Autodesk Fusion 360 part; units mm, degrees
(part 10 of 18)
  line L6698 (176.3253, -58.2178) -> (176.3253, -57.3778)
  line L6699 (176.3253, -57.3778) -> (177.2353, -57.3778)
  line L6700 (180.5454, -57.3778) -> (180.5454, -58.2178)
  line L6701 (180.5454, -58.2178) -> (179.6354, -58.2178)
  line L6702 (179.6354, -58.2178) -> (179.6354, -57.3778)
  line L6703 (179.6354, -57.3778) -> (180.5454, -57.3778)
  line L6704 (176.3253, -38.3151) -> (177.2353, -38.3151)
  line L6705 (177.2353, -39.1551) -> (176.3253, -39.1551)
  line L6706 (176.3253, -39.1551) -> (176.3253, -38.3151)
  line L6707 (177.2353, -38.3151) -> (177.2353, -39.1551)
  line L6708 (180.5454, -39.1551) -> (179.6354, -39.1551)
  line L6709 (180.5454, -38.3151) -> (180.5454, -39.1551)
  line L6710 (179.6354, -38.3151) -> (180.5454, -38.3151)
  line L6711 (179.6354, -39.1551) -> (179.6354, -38.3151)
  line L6712 (100.1251, -77.2806) -> (100.1251, -76.4406)
  line L6713 (100.1251, -76.4406) -> (101.0351, -76.4406)
  line L6714 (101.0351, -77.2806) -> (100.1251, -77.2806)
  line L6715 (101.0351, -76.4406) -> (101.0351, -77.2806)
  line L6716 (104.3453, -77.2806) -> (103.4353, -77.2806)
  line L6717 (104.3453, -76.4406) -> (104.3453, -77.2806)
  line L6718 (103.4353, -76.4406) -> (104.3453, -76.4406)
  line L6719 (103.4353, -77.2806) -> (103.4353, -76.4406)
  line L6720 (100.1251, -57.3778) -> (101.0351, -57.3778)
  line L6721 (101.0351, -58.2178) -> (100.1251, -58.2178)
  line L6722 (100.1251, -58.2178) -> (100.1251, -57.3778)
  line L6723 (101.0351, -57.3778) -> (101.0351, -58.2178)
  line L6724 (104.3453, -58.2178) -> (103.4353, -58.2178)
  line L6725 (104.3453, -57.3778) -> (104.3453, -58.2178)
  line L6726 (103.4353, -58.2178) -> (103.4353, -57.3778)
  line L6727 (103.4353, -57.3778) -> (104.3453, -57.3778)
  line L6728 (100.1251, -19.265) -> (101.0351, -19.265)
  line L6729 (101.0351, -20.105) -> (100.1251, -20.105)
  line L6730 (100.1251, -20.105) -> (100.1251, -19.265)
  line L6731 (101.0351, -19.265) -> (101.0351, -20.105)
  line L6732 (103.4353, -20.105) -> (103.4353, -19.265)
  line L6733 (104.3453, -20.105) -> (103.4353, -20.105)
  line L6734 (104.3453, -19.265) -> (104.3453, -20.105)
  line L6735 (103.4353, -19.265) -> (104.3453, -19.265)
  line L6736 (100.1251, -39.1551) -> (100.1251, -38.3151)
  line L6737 (100.1251, -38.3151) -> (101.0351, -38.3151)
  line L6738 (101.0351, -38.3151) -> (101.0351, -39.1551)
  line L6739 (101.0351, -39.1551) -> (100.1251, -39.1551)
  line L6740 (104.3453, -38.3151) -> (104.3453, -39.1551)
  line L6741 (103.4353, -39.1551) -> (103.4353, -38.3151)
  line L6742 (104.3453, -39.1551) -> (103.4353, -39.1551)
  line L6743 (103.4353, -38.3151) -> (104.3453, -38.3151)
  line L6744 (119.1752, -20.105) -> (119.1752, -19.265)
  line L6745 (120.0852, -20.105) -> (119.1752, -20.105)
  line L6746 (119.1752, -19.265) -> (120.0852, -19.265)
  line L6747 (120.0852, -19.265) -> (120.0852, -20.105)
  line L6748 (122.4853, -19.265) -> (123.3953, -19.265)
  line L6749 (123.3953, -20.105) -> (122.4853, -20.105)
  line L6750 (123.3953, -19.265) -> (123.3953, -20.105)
  line L6751 (122.4853, -20.105) -> (122.4853, -19.265)
  line L6752 (119.1752, -58.2178) -> (119.1752, -57.3778)
  line L6753 (120.0852, -58.2178) -> (119.1752, -58.2178)
  line L6754 (120.0852, -57.3778) -> (120.0852, -58.2178)
  line L6755 (119.1752, -57.3778) -> (120.0852, -57.3778)
  line L6756 (122.4853, -58.2178) -> (122.4853, -57.3778)
  line L6757 (123.3953, -57.3778) -> (123.3953, -58.2178)
  line L6758 (123.3953, -58.2178) -> (122.4853, -58.2178)
  line L6759 (122.4853, -57.3778) -> (123.3953, -57.3778)
  line L6760 (120.0852, -38.3151) -> (120.0852, -39.1551)
  line L6761 (119.1752, -38.3151) -> (120.0852, -38.3151)
  line L6762 (119.1752, -39.1551) -> (119.1752, -38.3151)
  line L6763 (120.0852, -39.1551) -> (119.1752, -39.1551)
  line L6764 (123.3953, -38.3151) -> (123.3953, -39.1551)
  line L6765 (123.3953, -39.1551) -> (122.4853, -39.1551)
  line L6766 (122.4853, -39.1551) -> (122.4853, -38.3151)
  line L6767 (122.4853, -38.3151) -> (123.3953, -38.3151)
  line L6768 (120.0852, -77.2806) -> (119.1752, -77.2806)
  line L6769 (119.1752, -77.2806) -> (119.1752, -76.4406)
  line L6770 (119.1752, -76.4406) -> (120.0852, -76.4406)
  line L6771 (120.0852, -76.4406) -> (120.0852, -77.2806)
  line L6772 (123.3953, -77.2806) -> (122.4853, -77.2806)
  line L6773 (123.3953, -76.4406) -> (123.3953, -77.2806)
  line L6774 (122.4853, -76.4406) -> (123.3953, -76.4406)
  line L6775 (122.4853, -77.2806) -> (122.4853, -76.4406)
  line L6776 (5.785, -76.4406) -> (5.785, -77.2806)
  line L6777 (5.785, -77.2806) -> (4.8749, -77.2806)
  line L6778 (4.8749, -76.4406) -> (5.785, -76.4406)
  line L6779 (4.8749, -77.2806) -> (4.8749, -76.4406)
  line L6780 (9.0951, -76.4406) -> (9.0951, -77.2806)
  line L6781 (8.1851, -76.4406) -> (9.0951, -76.4406)
  line L6782 (8.1851, -77.2806) -> (8.1851, -76.4406)
  line L6783 (9.0951, -77.2806) -> (8.1851, -77.2806)
  line L6784 (23.925, -76.4406) -> (24.835, -76.4406)
  line L6785 (23.925, -77.2806) -> (23.925, -76.4406)
  line L6786 (24.835, -77.2806) -> (23.925, -77.2806)
  line L6787 (24.835, -76.4406) -> (24.835, -77.2806)
  line L6788 (28.1451, -76.4406) -> (28.1451, -77.2806)
  line L6789 (28.1451, -77.2806) -> (27.2351, -77.2806)
  line L6790 (27.2351, -77.2806) -> (27.2351, -76.4406)
  line L6791 (27.2351, -76.4406) -> (28.1451, -76.4406)
  line L6792 (42.975, -76.4406) -> (43.885, -76.4406)
  line L6793 (42.975, -77.2806) -> (42.975, -76.4406)
  line L6794 (43.885, -77.2806) -> (42.975, -77.2806)
  line L6795 (43.885, -76.4406) -> (43.885, -77.2806)
  line L6796 (46.2852, -77.2806) -> (46.2852, -76.4406)
  line L6797 (47.1952, -76.4406) -> (47.1952, -77.2806)
  line L6798 (47.1952, -77.2806) -> (46.2852, -77.2806)
  line L6799 (46.2852, -76.4406) -> (47.1952, -76.4406)
  line L6800 (62.0251, -19.265) -> (62.9351, -19.265)
  line L6801 (62.0251, -20.105) -> (62.0251, -19.265)
  line L6802 (62.9351, -20.105) -> (62.0251, -20.105)
  line L6803 (62.9351, -19.265) -> (62.9351, -20.105)
  line L6804 (65.3352, -20.105) -> (65.3352, -19.265)
  line L6805 (65.3352, -19.265) -> (66.2452, -19.265)
  line L6806 (66.2452, -20.105) -> (65.3352, -20.105)
  line L6807 (66.2452, -19.265) -> (66.2452, -20.105)
  line L6808 (62.0251, -76.4406) -> (62.9351, -76.4406)
  line L6809 (62.0251, -77.2806) -> (62.0251, -76.4406)
  line L6810 (62.9351, -76.4406) -> (62.9351, -77.2806)
  line L6811 (62.9351, -77.2806) -> (62.0251, -77.2806)
  line L6812 (65.3352, -76.4406) -> (66.2452, -76.4406)
  line L6813 (66.2452, -76.4406) -> (66.2452, -77.2806)
  line L6814 (66.2452, -77.2806) -> (65.3352, -77.2806)
  line L6815 (65.3352, -77.2806) -> (65.3352, -76.4406)
  line L6816 (62.0251, -38.3151) -> (62.9351, -38.3151)
  line L6817 (62.9351, -38.3151) -> (62.9351, -39.1551)
  line L6818 (62.0251, -39.1551) -> (62.0251, -38.3151)
  line L6819 (62.9351, -39.1551) -> (62.0251, -39.1551)
  line L6820 (66.2452, -38.3151) -> (66.2452, -39.1551)
  line L6821 (66.2452, -39.1551) -> (65.3352, -39.1551)
  line L6822 (65.3352, -38.3151) -> (66.2452, -38.3151)
  line L6823 (65.3352, -39.1551) -> (65.3352, -38.3151)
  line L6824 (62.9351, -58.2178) -> (62.0251, -58.2178)
  line L6825 (62.0251, -57.3778) -> (62.9351, -57.3778)
  line L6826 (62.0251, -58.2178) -> (62.0251, -57.3778)
  line L6827 (62.9351, -57.3778) -> (62.9351, -58.2178)
  line L6828 (66.2452, -57.3778) -> (66.2452, -58.2178)
  line L6829 (65.3352, -57.3778) -> (66.2452, -57.3778)
  line L6830 (66.2452, -58.2178) -> (65.3352, -58.2178)
  line L6831 (65.3352, -58.2178) -> (65.3352, -57.3778)
  line L6832 (81.9851, -39.1551) -> (81.0751, -39.1551)
  line L6833 (81.0751, -38.3151) -> (81.9851, -38.3151)
  line L6834 (81.9851, -38.3151) -> (81.9851, -39.1551)
  line L6835 (81.0751, -39.1551) -> (81.0751, -38.3151)
  line L6836 (84.3852, -38.3151) -> (85.2952, -38.3151)
  line L6837 (85.2952, -39.1551) -> (84.3852, -39.1551)
  line L6838 (84.3852, -39.1551) -> (84.3852, -38.3151)
  line L6839 (85.2952, -38.3151) -> (85.2952, -39.1551)
  line L6840 (81.9851, -77.2806) -> (81.0751, -77.2806)
  line L6841 (81.9851, -76.4406) -> (81.9851, -77.2806)
  line L6842 (81.0751, -77.2806) -> (81.0751, -76.4406)
  line L6843 (81.0751, -76.4406) -> (81.9851, -76.4406)
  line L6844 (84.3852, -76.4406) -> (85.2952, -76.4406)
  line L6845 (85.2952, -77.2806) -> (84.3852, -77.2806)
  line L6846 (84.3852, -77.2806) -> (84.3852, -76.4406)
  line L6847 (85.2952, -76.4406) -> (85.2952, -77.2806)
  line L6848 (81.9851, -19.265) -> (81.9851, -20.105)
  line L6849 (81.9851, -20.105) -> (81.0751, -20.105)
  line L6850 (81.0751, -19.265) -> (81.9851, -19.265)
  line L6851 (81.0751, -20.105) -> (81.0751, -19.265)
  line L6852 (85.2952, -19.265) -> (85.2952, -20.105)
  line L6853 (84.3852, -19.265) -> (85.2952, -19.265)
  line L6854 (84.3852, -20.105) -> (84.3852, -19.265)
  line L6855 (85.2952, -20.105) -> (84.3852, -20.105)
  line L6856 (81.9851, -58.2178) -> (81.0751, -58.2178)
  line L6857 (81.0751, -57.3778) -> (81.9851, -57.3778)
  line L6858 (81.9851, -57.3778) -> (81.9851, -58.2178)
  line L6859 (81.0751, -58.2178) -> (81.0751, -57.3778)
  line L6860 (84.3852, -58.2178) -> (84.3852, -57.3778)
  line L6861 (85.2952, -57.3778) -> (85.2952, -58.2178)
  line L6862 (84.3852, -57.3778) -> (85.2952, -57.3778)
  line L6863 (85.2952, -58.2178) -> (84.3852, -58.2178)
  line L6864 (5.785, -58.2178) -> (4.8749, -58.2178)
  line L6865 (5.785, -57.3778) -> (5.785, -58.2178)
  line L6866 (4.8749, -57.3778) -> (5.785, -57.3778)
  line L6867 (4.8749, -58.2178) -> (4.8749, -57.3778)
  line L6868 (8.1851, -58.2178) -> (8.1851, -57.3778)
  line L6869 (8.1851, -57.3778) -> (9.0951, -57.3778)
  line L6870 (9.0951, -57.3778) -> (9.0951, -58.2178)
  line L6871 (9.0951, -58.2178) -> (8.1851, -58.2178)
  line L6872 (4.8749, -19.265) -> (5.785, -19.265)
  line L6873 (5.785, -20.105) -> (4.8749, -20.105)
  line L6874 (5.785, -19.265) -> (5.785, -20.105)
  line L6875 (4.8749, -20.105) -> (4.8749, -19.265)
  line L6876 (8.1851, -20.105) -> (8.1851, -19.265)
  line L6877 (9.0951, -20.105) -> (8.1851, -20.105)
  line L6878 (8.1851, -19.265) -> (9.0951, -19.265)
  line L6879 (9.0951, -19.265) -> (9.0951, -20.105)
  line L6880 (4.8749, -39.1551) -> (4.8749, -38.3151)
  line L6881 (5.785, -38.3151) -> (5.785, -39.1551)
  line L6882 (5.785, -39.1551) -> (4.8749, -39.1551)
  line L6883 (4.8749, -38.3151) -> (5.785, -38.3151)
  line L6884 (9.0951, -38.3151) -> (9.0951, -39.1551)
  line L6885 (8.1851, -39.1551) -> (8.1851, -38.3151)
  line L6886 (9.0951, -39.1551) -> (8.1851, -39.1551)
  line L6887 (8.1851, -38.3151) -> (9.0951, -38.3151)
  line L6888 (24.835, -38.3151) -> (24.835, -39.1551)
  line L6889 (24.835, -39.1551) -> (23.925, -39.1551)
  line L6890 (23.925, -39.1551) -> (23.925, -38.3151)
  line L6891 (23.925, -38.3151) -> (24.835, -38.3151)
  line L6892 (27.2351, -39.1551) -> (27.2351, -38.3151)
  line L6893 (28.1451, -39.1551) -> (27.2351, -39.1551)
  line L6894 (27.2351, -38.3151) -> (28.1451, -38.3151)
  line L6895 (28.1451, -38.3151) -> (28.1451, -39.1551)
  line L6896 (24.835, -19.265) -> (24.835, -20.105)
  line L6897 (23.925, -20.105) -> (23.925, -19.265)
  line L6898 (24.835, -20.105) -> (23.925, -20.105)
  line L6899 (23.925, -19.265) -> (24.835, -19.265)
  line L6900 (27.2351, -20.105) -> (27.2351, -19.265)
  line L6901 (28.1451, -19.265) -> (28.1451, -20.105)
  line L6902 (28.1451, -20.105) -> (27.2351, -20.105)
  line L6903 (27.2351, -19.265) -> (28.1451, -19.265)
  line L6904 (23.925, -58.2178) -> (23.925, -57.3778)
  line L6905 (24.835, -58.2178) -> (23.925, -58.2178)
  line L6906 (23.925, -57.3778) -> (24.835, -57.3778)
  line L6907 (24.835, -57.3778) -> (24.835, -58.2178)
  line L6908 (28.1451, -58.2178) -> (27.2351, -58.2178)
  line L6909 (28.1451, -57.3778) -> (28.1451, -58.2178)
  line L6910 (27.2351, -57.3778) -> (28.1451, -57.3778)
  line L6911 (27.2351, -58.2178) -> (27.2351, -57.3778)
  line L6912 (43.885, -19.265) -> (43.885, -20.105)
  line L6913 (42.975, -19.265) -> (43.885, -19.265)
  line L6914 (42.975, -20.105) -> (42.975, -19.265)
  line L6915 (43.885, -20.105) -> (42.975, -20.105)
  line L6916 (47.1952, -20.105) -> (46.2852, -20.105)
  line L6917 (47.1952, -19.265) -> (47.1952, -20.105)
  line L6918 (46.2852, -19.265) -> (47.1952, -19.265)
  line L6919 (46.2852, -20.105) -> (46.2852, -19.265)
  line L6920 (43.885, -57.3778) -> (43.885, -58.2178)
  line L6921 (42.975, -57.3778) -> (43.885, -57.3778)
  line L6922 (42.975, -58.2178) -> (42.975, -57.3778)
  line L6923 (43.885, -58.2178) -> (42.975, -58.2178)
  line L6924 (46.2852, -57.3778) -> (47.1952, -57.3778)
  line L6925 (47.1952, -57.3778) -> (47.1952, -58.2178)
  line L6926 (46.2852, -58.2178) -> (46.2852, -57.3778)
  line L6927 (47.1952, -58.2178) -> (46.2852, -58.2178)
  line L6928 (43.885, -38.3151) -> (43.885, -39.1551)
  line L6929 (42.975, -38.3151) -> (43.885, -38.3151)
  line L6930 (43.885, -39.1551) -> (42.975, -39.1551)
  line L6931 (42.975, -39.1551) -> (42.975, -38.3151)
  line L6932 (47.1952, -38.3151) -> (47.1952, -39.1551)
  line L6933 (46.2852, -39.1551) -> (46.2852, -38.3151)
  line L6934 (47.1952, -39.1551) -> (46.2852, -39.1551)
  line L6935 (46.2852, -38.3151) -> (47.1952, -38.3151)
  line L6936 (215.3354, -20.105) -> (214.4254, -20.105)
  line L6937 (214.4254, -19.265) -> (215.3354, -19.265)
  line L6938 (214.4254, -20.105) -> (214.4254, -19.265)
  line L6939 (215.3354, -19.265) -> (215.3354, -20.105)
  line L6940 (218.6455, -19.265) -> (218.6455, -20.105)
  line L6941 (217.7355, -20.105) -> (217.7355, -19.265)
  line L6942 (218.6455, -20.105) -> (217.7355, -20.105)
  line L6943 (217.7355, -19.265) -> (218.6455, -19.265)
  line L6944 (215.3354, -76.4406) -> (215.3354, -77.2806)
  line L6945 (214.4254, -76.4406) -> (215.3354, -76.4406)
  line L6946 (214.4254, -77.2806) -> (214.4254, -76.4406)
  line L6947 (215.3354, -77.2806) -> (214.4254, -77.2806)
  line L6948 (218.6455, -77.2806) -> (217.7355, -77.2806)
  line L6949 (217.7355, -77.2806) -> (217.7355, -76.4406)
  line L6950 (218.6455, -76.4406) -> (218.6455, -77.2806)
  line L6951 (217.7355, -76.4406) -> (218.6455, -76.4406)
  line L6952 (214.4254, -57.3778) -> (215.3354, -57.3778)
  line L6953 (214.4254, -58.2178) -> (214.4254, -57.3778)
  line L6954 (215.3354, -58.2178) -> (214.4254, -58.2178)
  line L6955 (215.3354, -57.3778) -> (215.3354, -58.2178)
  line L6956 (217.7355, -58.2178) -> (217.7355, -57.3778)
  line L6957 (217.7355, -57.3778) -> (218.6455, -57.3778)
  line L6958 (218.6455, -58.2178) -> (217.7355, -58.2178)
  line L6959 (218.6455, -57.3778) -> (218.6455, -58.2178)
  line L6960 (214.4254, -38.3151) -> (215.3354, -38.3151)
  line L6961 (214.4254, -39.1551) -> (214.4254, -38.3151)
  line L6962 (215.3354, -39.1551) -> (214.4254, -39.1551)
  line L6963 (215.3354, -38.3151) -> (215.3354, -39.1551)
  line L6964 (217.7355, -39.1551) -> (217.7355, -38.3151)
  line L6965 (218.6455, -38.3151) -> (218.6455, -39.1551)
  line L6966 (218.6455, -39.1551) -> (217.7355, -39.1551)
  line L6967 (217.7355, -38.3151) -> (218.6455, -38.3151)
  line L6968 (196.2853, -38.3151) -> (196.2853, -39.1551)
  line L6969 (195.3753, -39.1551) -> (195.3753, -38.3151)
  line L6970 (196.2853, -39.1551) -> (195.3753, -39.1551)
  line L6971 (195.3753, -38.3151) -> (196.2853, -38.3151)
  line L6972 (199.5955, -38.3151) -> (199.5955, -39.1551)
  line L6973 (198.6855, -39.1551) -> (198.6855, -38.3151)
  line L6974 (199.5955, -39.1551) -> (198.6855, -39.1551)
  line L6975 (198.6855, -38.3151) -> (199.5955, -38.3151)
  line L6976 (195.3753, -76.4406) -> (196.2853, -76.4406)
  line L6977 (196.2853, -76.4406) -> (196.2853, -77.2806)
  line L6978 (196.2853, -77.2806) -> (195.3753, -77.2806)
  line L6979 (195.3753, -77.2806) -> (195.3753, -76.4406)
  line L6980 (199.5955, -77.2806) -> (198.6855, -77.2806)
  line L6981 (198.6855, -76.4406) -> (199.5955, -76.4406)
  line L6982 (198.6855, -77.2806) -> (198.6855, -76.4406)
  line L6983 (199.5955, -76.4406) -> (199.5955, -77.2806)
  line L6984 (196.2853, -58.2178) -> (195.3753, -58.2178)
  line L6985 (195.3753, -57.3778) -> (196.2853, -57.3778)
  line L6986 (195.3753, -58.2178) -> (195.3753, -57.3778)
  line L6987 (196.2853, -57.3778) -> (196.2853, -58.2178)
  line L6988 (199.5955, -57.3778) -> (199.5955, -58.2178)
  line L6989 (198.6855, -58.2178) -> (198.6855, -57.3778)
  line L6990 (198.6855, -57.3778) -> (199.5955, -57.3778)
  line L6991 (199.5955, -58.2178) -> (198.6855, -58.2178)
  line L6992 (196.2853, -19.265) -> (196.2853, -20.105)
  line L6993 (195.3753, -20.105) -> (195.3753, -19.265)
  line L6994 (196.2853, -20.105) -> (195.3753, -20.105)
  line L6995 (195.3753, -19.265) -> (196.2853, -19.265)
  line L6996 (199.5955, -19.265) -> (199.5955, -20.105)
  line L6997 (198.6855, -20.105) -> (198.6855, -19.265)
  line L6998 (198.6855, -19.265) -> (199.5955, -19.265)
  line L6999 (199.5955, -20.105) -> (198.6855, -20.105)
  line L7000 (202.1384, -4.26) -> (201.3384, -4.26)
  line L7001 (202.1384, -3.36) -> (202.1384, -4.26)
  line L7002 (201.3384, -3.36) -> (202.1384, -3.36)
  line L7003 (201.3384, -4.26) -> (201.3384, -3.36)
  line L7004 (202.7384, -3.36) -> (203.5384, -3.36)
  line L7005 (203.5384, -3.36) -> (203.5384, -4.26)
  line L7006 (202.7384, -4.26) -> (202.7384, -3.36)
  line L7007 (203.5384, -4.26) -> (202.7384, -4.26)
  line L7008 (200.2334, -6.281) -> (200.2334, -7.181)
  line L7009 (200.2334, -7.181) -> (199.4334, -7.181)
  line L7010 (199.4334, -6.281) -> (200.2334, -6.281)
  line L7011 (199.4334, -7.181) -> (199.4334, -6.281)
  line L7012 (201.6334, -7.181) -> (200.8334, -7.181)
  line L7013 (200.8334, -6.281) -> (201.6334, -6.281)
  line L7014 (201.6334, -6.281) -> (201.6334, -7.181)
  line L7015 (200.8334, -7.181) -> (200.8334, -6.281)
  line L7016 (206.8404, -4.376) -> (206.8404, -5.276)
  line L7017 (206.8404, -5.276) -> (206.0404, -5.276)
  line L7018 (206.0404, -4.376) -> (206.8404, -4.376)
  line L7019 (206.0404, -5.276) -> (206.0404, -4.376)
  line L7020 (205.4404, -4.376) -> (205.4404, -5.276)
  line L7021 (204.6404, -5.276) -> (204.6404, -4.376)
  line L7022 (204.6404, -4.376) -> (205.4404, -4.376)
  line L7023 (205.4404, -5.276) -> (204.6404, -5.276)
  arc A868 (8.7631, -8.0011) -> (10.5631, -8.0011) centre (9.6631, -8.0011) ccw
  arc A869 (10.5631, -8.0011) -> (8.7631, -8.0011) centre (9.6631, -8.0011) ccw
  arc A870 (10.5631, -5.4611) -> (8.7631, -5.4611) centre (9.6631, -5.4611) ccw
  arc A871 (8.7631, -5.4611) -> (10.5631, -5.4611) centre (9.6631, -5.4611) ccw
  arc A872 (8.7631, -2.9211) -> (10.5631, -2.9211) centre (9.6631, -2.9211) ccw
  arc A873 (10.5631, -2.9211) -> (8.7631, -2.9211) centre (9.6631, -2.9211) ccw
  arc A874 (-3.9371, -8.0011) -> (-5.7371, -8.0011) centre (-4.8371, -8.0011) ccw
  arc A875 (-5.7371, -8.0011) -> (-3.9371, -8.0011) centre (-4.8371, -8.0011) ccw
  line L7024 (-3.9371, -8.0011) -> (-3.9371, -8.0011)
  arc A876 (-3.9371, -2.9211) -> (-5.7371, -2.9211) centre (-4.8371, -2.9211) ccw
  arc A877 (-5.7371, -2.9211) -> (-3.9371, -2.9211) centre (-4.8371, -2.9211) ccw
  line L7025 (-3.9371, -2.9211) -> (-3.9371, -2.9211)
  line L7026 (3.8261, 0.8522) -> (4.0754, 0.4791)
  line L7027 (0.2505, -0.4011) -> (0.1629, 0.039)
  line L7028 (0.1629, 0.039) -> (0.2505, 0.4791)
  line L7029 (0.4998, 0.8522) -> (0.8729, 1.1015)
  line L7030 (4.0754, 0.4791) -> (4.1629, 0.039)
  line L7031 (1.3129, -1.111) -> (0.8729, -1.0235)
  line L7032 (3.8261, -0.7742) -> (3.453, -1.0235)
  line L7033 (3.0129, 1.189) -> (3.453, 1.1015)
  line L7034 (0.4998, -0.7742) -> (0.2505, -0.4011)
  line L7035 (3.453, 1.1015) -> (3.8261, 0.8522)
  line L7036 (1.3129, 1.189) -> (3.0129, 1.189)
  line L7037 (0.2505, 0.4791) -> (0.4998, 0.8522)
  line L7038 (4.0754, -0.4011) -> (3.8261, -0.7742)
  line L7039 (3.0129, -1.111) -> (1.3129, -1.111)
  line L7040 (0.8729, -1.0235) -> (0.4998, -0.7742)
  line L7041 (4.1629, 0.039) -> (4.0754, -0.4011)
  line L7042 (3.453, -1.0235) -> (3.0129, -1.111)
  line L7043 (0.8729, 1.1015) -> (1.3129, 1.189)
  line L7044 (3.453, -9.8985) -> (3.8261, -10.1478)
  line L7045 (0.8729, -12.0235) -> (0.4998, -11.7742)
  line L7046 (0.1629, -10.961) -> (0.2505, -10.5209)
  line L7047 (3.8261, -11.7742) -> (3.453, -12.0235)
  line L7048 (0.4998, -10.1478) -> (0.8729, -9.8985)
  line L7049 (0.4998, -11.7742) -> (0.2505, -11.4011)
  line L7050 (4.0754, -10.5209) -> (4.1629, -10.961)
  line L7051 (1.3129, -12.111) -> (0.8729, -12.0235)
  line L7052 (4.1629, -10.961) -> (4.0754, -11.4011)
  line L7053 (3.8261, -10.1478) -> (4.0754, -10.5209)
  line L7054 (0.2505, -10.5209) -> (0.4998, -10.1478)
  line L7055 (3.0129, -9.811) -> (3.453, -9.8985)
  line L7056 (0.8729, -9.8985) -> (1.3129, -9.811)
  line L7057 (1.3129, -9.811) -> (3.0129, -9.811)
  line L7058 (0.2505, -11.4011) -> (0.1629, -10.961)
  line L7059 (4.0754, -11.4011) -> (3.8261, -11.7742)
  line L7060 (3.453, -12.0235) -> (3.0129, -12.111)
  line L7061 (3.0129, -12.111) -> (1.3129, -12.111)
  line L7062 (195.5924, -3.595) -> (195.5924, -3.995)
  line L7063 (194.7924, -3.595) -> (195.5924, -3.595)
  line L7064 (195.5924, -3.995) -> (194.7924, -3.995)
  line L7065 (194.7924, -3.995) -> (194.7924, -3.595)
  line L7066 (194.7924, -4.645) -> (194.7924, -4.245)
  line L7067 (194.7924, -4.245) -> (195.5924, -4.245)
  line L7068 (195.5924, -4.245) -> (195.5924, -4.645)
  line L7069 (195.5924, -4.645) -> (194.7924, -4.645)
  line L7070 (194.7924, -5.295) -> (194.7924, -4.895)
  line L7071 (195.5924, -5.295) -> (194.7924, -5.295)
  line L7072 (195.5924, -4.895) -> (195.5924, -5.295)
  line L7073 (194.7924, -4.895) -> (195.5924, -4.895)
  line L7074 (197.8924, -4.895) -> (197.8924, -5.295)
  line L7075 (197.0924, -5.295) -> (197.0924, -4.895)
  line L7076 (197.0924, -4.895) -> (197.8924, -4.895)
  line L7077 (197.8924, -5.295) -> (197.0924, -5.295)
  line L7078 (197.8924, -3.995) -> (197.0924, -3.995)
  line L7079 (197.8924, -3.595) -> (197.8924, -3.995)
  line L7080 (197.0924, -3.995) -> (197.0924, -3.595)
  line L7081 (197.0924, -3.595) -> (197.8924, -3.595)
  arc A878 (194.7974, -61.2644) -> (195.9974, -61.2644) centre (195.3974, -61.2644) ccw
  arc A879 (195.9974, -61.2644) -> (194.7974, -61.2644) centre (195.3974, -61.2644) ccw
  arc A880 (191.2974, -63.5184) -> (192.4974, -63.5184) centre (191.8974, -63.5184) ccw
  arc A881 (192.4974, -63.5184) -> (191.2974, -63.5184) centre (191.8974, -63.5184) ccw
  arc A882 (176.9474, -80.3272) -> (175.7474, -80.3272) centre (176.3474, -80.3272) ccw
  arc A883 (175.7474, -80.3272) -> (176.9474, -80.3272) centre (176.3474, -80.3272) ccw
  arc A884 (173.4473, -82.5812) -> (172.2473, -82.5812) centre (172.8473, -82.5812) ccw
  arc A885 (172.2473, -82.5812) -> (173.4473, -82.5812) centre (172.8473, -82.5812) ccw
  arc A886 (176.9474, -61.2644) -> (175.7474, -61.2644) centre (176.3474, -61.2644) ccw
  arc A887 (175.7474, -61.2644) -> (176.9474, -61.2644) centre (176.3474, -61.2644) ccw
  arc A888 (173.4473, -63.5184) -> (172.2473, -63.5184) centre (172.8473, -63.5184) ccw
  arc A889 (172.2473, -63.5184) -> (173.4473, -63.5184) centre (172.8473, -63.5184) ccw
  arc A890 (175.7474, -42.2017) -> (176.9474, -42.2017) centre (176.3474, -42.2017) ccw
  arc A891 (176.9474, -42.2017) -> (175.7474, -42.2017) centre (176.3474, -42.2017) ccw
  arc A892 (172.2473, -44.4557) -> (173.4473, -44.4557) centre (172.8473, -44.4557) ccw
  arc A893 (173.4473, -44.4557) -> (172.2473, -44.4557) centre (172.8473, -44.4557) ccw
  arc A894 (176.9474, -23.1516) -> (175.7474, -23.1516) centre (176.3474, -23.1516) ccw
  arc A895 (175.7474, -23.1516) -> (176.9474, -23.1516) centre (176.3474, -23.1516) ccw
  arc A896 (173.4473, -25.4057) -> (172.2473, -25.4057) centre (172.8473, -25.4057) ccw
  arc A897 (172.2473, -25.4057) -> (173.4473, -25.4057) centre (172.8473, -25.4057) ccw
  arc A898 (157.8973, -80.3272) -> (156.6973, -80.3272) centre (157.2973, -80.3272) ccw
  arc A899 (156.6973, -80.3272) -> (157.8973, -80.3272) centre (157.2973, -80.3272) ccw
  arc A900 (154.3973, -82.5812) -> (153.1973, -82.5812) centre (153.7973, -82.5812) ccw
  arc A901 (153.1973, -82.5812) -> (154.3973, -82.5812) centre (153.7973, -82.5812) ccw
  arc A902 (156.6973, -42.2017) -> (157.8973, -42.2017) centre (157.2973, -42.2017) ccw
  arc A903 (157.8973, -42.2017) -> (156.6973, -42.2017) centre (157.2973, -42.2017) ccw
  arc A904 (153.1973, -44.4557) -> (154.3973, -44.4557) centre (153.7973, -44.4557) ccw
  arc A905 (154.3973, -44.4557) -> (153.1973, -44.4557) centre (153.7973, -44.4557) ccw
  arc A906 (157.8973, -61.2644) -> (156.6973, -61.2644) centre (157.2973, -61.2644) ccw
  arc A907 (156.6973, -61.2644) -> (157.8973, -61.2644) centre (157.2973, -61.2644) ccw
  arc A908 (153.1973, -63.5184) -> (154.3973, -63.5184) centre (153.7973, -63.5184) ccw
  arc A909 (154.3973, -63.5184) -> (153.1973, -63.5184) centre (153.7973, -63.5184) ccw
  arc A910 (157.8973, -23.1516) -> (156.6973, -23.1516) centre (157.2973, -23.1516) ccw
  arc A911 (156.6973, -23.1516) -> (157.8973, -23.1516) centre (157.2973, -23.1516) ccw
  arc A912 (154.3973, -25.4057) -> (153.1973, -25.4057) centre (153.7973, -25.4057) ccw
  arc A913 (153.1973, -25.4057) -> (154.3973, -25.4057) centre (153.7973, -25.4057) ccw
  arc A914 (137.6473, -61.2644) -> (138.8473, -61.2644) centre (138.2473, -61.2644) ccw
  arc A915 (138.8473, -61.2644) -> (137.6473, -61.2644) centre (138.2473, -61.2644) ccw
  arc A916 (135.3473, -63.5184) -> (134.1473, -63.5184) centre (134.7473, -63.5184) ccw
  arc A917 (134.1473, -63.5184) -> (135.3473, -63.5184) centre (134.7473, -63.5184) ccw
  arc A918 (138.8473, -42.2017) -> (137.6473, -42.2017) centre (138.2473, -42.2017) ccw
  arc A919 (137.6473, -42.2017) -> (138.8473, -42.2017) centre (138.2473, -42.2017) ccw
  arc A920 (135.3473, -44.4557) -> (134.1473, -44.4557) centre (134.7473, -44.4557) ccw
  arc A921 (134.1473, -44.4557) -> (135.3473, -44.4557) centre (134.7473, -44.4557) ccw
  arc A922 (137.6473, -23.1516) -> (138.8473, -23.1516) centre (138.2473, -23.1516) ccw
  arc A923 (138.8473, -23.1516) -> (137.6473, -23.1516) centre (138.2473, -23.1516) ccw
  arc A924 (134.1473, -25.4057) -> (135.3473, -25.4057) centre (134.7473, -25.4057) ccw
  arc A925 (135.3473, -25.4057) -> (134.1473, -25.4057) centre (134.7473, -25.4057) ccw
  arc A926 (138.8473, -80.3272) -> (137.6473, -80.3272) centre (138.2473, -80.3272) ccw
  arc A927 (137.6473, -80.3272) -> (138.8473, -80.3272) centre (138.2473, -80.3272) ccw
  arc A928 (135.3473, -82.5812) -> (134.1473, -82.5812) centre (134.7473, -82.5812) ccw
  arc A929 (134.1473, -82.5812) -> (135.3473, -82.5812) centre (134.7473, -82.5812) ccw
  arc A930 (119.7972, -80.3272) -> (118.5972, -80.3272) centre (119.1972, -80.3272) ccw
  arc A931 (118.5972, -80.3272) -> (119.7972, -80.3272) centre (119.1972, -80.3272) ccw
  arc A932 (115.0972, -82.5812) -> (116.2972, -82.5812) centre (115.6972, -82.5812) ccw
  arc A933 (116.2972, -82.5812) -> (115.0972, -82.5812) centre (115.6972, -82.5812) ccw
  arc A934 (119.7972, -61.2644) -> (118.5972, -61.2644) centre (119.1972, -61.2644) ccw
  arc A935 (118.5972, -61.2644) -> (119.7972, -61.2644) centre (119.1972, -61.2644) ccw
  arc A936 (115.0972, -63.5184) -> (116.2972, -63.5184) centre (115.6972, -63.5184) ccw
  arc A937 (116.2972, -63.5184) -> (115.0972, -63.5184) centre (115.6972, -63.5184) ccw
  arc A938 (119.7972, -23.1516) -> (118.5972, -23.1516) centre (119.1972, -23.1516) ccw
  arc A939 (118.5972, -23.1516) -> (119.7972, -23.1516) centre (119.1972, -23.1516) ccw
  arc A940 (115.0972, -25.4057) -> (116.2972, -25.4057) centre (115.6972, -25.4057) ccw
  arc A941 (116.2972, -25.4057) -> (115.0972, -25.4057) centre (115.6972, -25.4057) ccw
  arc A942 (118.5972, -42.2017) -> (119.7972, -42.2017) centre (119.1972, -42.2017) ccw
  arc A943 (119.7972, -42.2017) -> (118.5972, -42.2017) centre (119.1972, -42.2017) ccw
  arc A944 (116.2972, -44.4557) -> (115.0972, -44.4557) centre (115.6972, -44.4557) ccw
  arc A945 (115.0972, -44.4557) -> (116.2972, -44.4557) centre (115.6972, -44.4557) ccw
  arc A946 (100.7472, -23.1516) -> (99.5472, -23.1516) centre (100.1472, -23.1516) ccw
  arc A947 (99.5472, -23.1516) -> (100.7472, -23.1516) centre (100.1472, -23.1516) ccw
  arc A948 (97.2472, -25.4057) -> (96.0472, -25.4057) centre (96.6472, -25.4057) ccw
  arc A949 (96.0472, -25.4057) -> (97.2472, -25.4057) centre (96.6472, -25.4057) ccw
  arc A950 (99.5472, -42.2017) -> (100.7472, -42.2017) centre (100.1472, -42.2017) ccw
  arc A951 (100.7472, -42.2017) -> (99.5472, -42.2017) centre (100.1472, -42.2017) ccw
  arc A952 (96.0472, -44.4557) -> (97.2472, -44.4557) centre (96.6472, -44.4557) ccw
  arc A953 (97.2472, -44.4557) -> (96.0472, -44.4557) centre (96.6472, -44.4557) ccw
  arc A954 (100.7472, -80.3272) -> (99.5472, -80.3272) centre (100.1472, -80.3272) ccw
  arc A955 (99.5472, -80.3272) -> (100.7472, -80.3272) centre (100.1472, -80.3272) ccw
  arc A956 (97.2472, -82.5812) -> (96.0472, -82.5812) centre (96.6472, -82.5812) ccw
  arc A957 (96.0472, -82.5812) -> (97.2472, -82.5812) centre (96.6472, -82.5812) ccw
  arc A958 (100.7472, -61.2644) -> (99.5472, -61.2644) centre (100.1472, -61.2644) ccw
  arc A959 (99.5472, -61.2644) -> (100.7472, -61.2644) centre (100.1472, -61.2644) ccw
  arc A960 (97.2472, -63.5184) -> (96.0472, -63.5184) centre (96.6472, -63.5184) ccw
  arc A961 (96.0472, -63.5184) -> (97.2472, -63.5184) centre (96.6472, -63.5184) ccw
  arc A962 (194.7974, -80.3272) -> (195.9974, -80.3272) centre (195.3974, -80.3272) ccw
  arc A963 (195.9974, -80.3272) -> (194.7974, -80.3272) centre (195.3974, -80.3272) ccw
  arc A964 (192.4974, -82.5812) -> (191.2974, -82.5812) centre (191.8974, -82.5812) ccw
  arc A965 (191.2974, -82.5812) -> (192.4974, -82.5812) centre (191.8974, -82.5812) ccw
  arc A966 (194.7974, -23.1516) -> (195.9974, -23.1516) centre (195.3974, -23.1516) ccw
  arc A967 (195.9974, -23.1516) -> (194.7974, -23.1516) centre (195.3974, -23.1516) ccw
  arc A968 (191.2974, -25.4057) -> (192.4974, -25.4057) centre (191.8974, -25.4057) ccw
  arc A969 (192.4974, -25.4057) -> (191.2974, -25.4057) centre (191.8974, -25.4057) ccw
  arc A970 (81.6972, -80.3272) -> (80.4972, -80.3272) centre (81.0972, -80.3272) ccw
  arc A971 (80.4972, -80.3272) -> (81.6972, -80.3272) centre (81.0972, -80.3272) ccw
  arc A972 (76.9972, -82.5812) -> (78.1972, -82.5812) centre (77.5972, -82.5812) ccw
  arc A973 (78.1972, -82.5812) -> (76.9972, -82.5812) centre (77.5972, -82.5812) ccw
  arc A974 (81.6972, -42.2017) -> (80.4972, -42.2017) centre (81.0972, -42.2017) ccw
  arc A975 (80.4972, -42.2017) -> (81.6972, -42.2017) centre (81.0972, -42.2017) ccw
  arc A976 (76.9972, -44.4557) -> (78.1972, -44.4557) centre (77.5972, -44.4557) ccw
  arc A977 (78.1972, -44.4557) -> (76.9972, -44.4557) centre (77.5972, -44.4557) ccw
  arc A978 (81.6972, -23.1516) -> (80.4972, -23.1516) centre (81.0972, -23.1516) ccw
  arc A979 (80.4972, -23.1516) -> (81.6972, -23.1516) centre (81.0972, -23.1516) ccw
  arc A980 (76.9972, -25.4057) -> (78.1972, -25.4057) centre (77.5972, -25.4057) ccw
  arc A981 (78.1972, -25.4057) -> (76.9972, -25.4057) centre (77.5972, -25.4057) ccw
  arc A982 (81.6972, -61.2644) -> (80.4972, -61.2644) centre (81.0972, -61.2644) ccw
  arc A983 (80.4972, -61.2644) -> (81.6972, -61.2644) centre (81.0972, -61.2644) ccw
  arc A984 (76.9972, -63.5184) -> (78.1972, -63.5184) centre (77.5972, -63.5184) ccw
  arc A985 (78.1972, -63.5184) -> (76.9972, -63.5184) centre (77.5972, -63.5184) ccw
  arc A986 (62.6471, -80.3272) -> (61.4471, -80.3272) centre (62.0471, -80.3272) ccw
  arc A987 (61.4471, -80.3272) -> (62.6471, -80.3272) centre (62.0471, -80.3272) ccw
  arc A988 (59.1471, -82.5812) -> (57.9471, -82.5812) centre (58.5471, -82.5812) ccw
  arc A989 (57.9471, -82.5812) -> (59.1471, -82.5812) centre (58.5471, -82.5812) ccw
  arc A990 (61.4471, -61.2644) -> (62.6471, -61.2644) centre (62.0471, -61.2644) ccw
  arc A991 (62.6471, -61.2644) -> (61.4471, -61.2644) centre (62.0471, -61.2644) ccw
  arc A992 (59.1471, -63.5184) -> (57.9471, -63.5184) centre (58.5471, -63.5184) ccw
  arc A993 (57.9471, -63.5184) -> (59.1471, -63.5184) centre (58.5471, -63.5184) ccw
  arc A994 (62.6471, -42.2017) -> (61.4471, -42.2017) centre (62.0471, -42.2017) ccw
  arc A995 (61.4471, -42.2017) -> (62.6471, -42.2017) centre (62.0471, -42.2017) ccw
  arc A996 (59.1471, -44.4557) -> (57.9471, -44.4557) centre (58.5471, -44.4557) ccw
  arc A997 (57.9471, -44.4557) -> (59.1471, -44.4557) centre (58.5471, -44.4557) ccw
  arc A998 (43.5971, -61.2644) -> (42.3971, -61.2644) centre (42.9971, -61.2644) ccw
  arc A999 (42.3971, -61.2644) -> (43.5971, -61.2644) centre (42.9971, -61.2644) ccw
  arc A1000 (38.8971, -63.5184) -> (40.0971, -63.5184) centre (39.4971, -63.5184) ccw
  arc A1001 (40.0971, -63.5184) -> (38.8971, -63.5184) centre (39.4971, -63.5184) ccw
  arc A1002 (43.5971, -80.3272) -> (42.3971, -80.3272) centre (42.9971, -80.3272) ccw
  arc A1003 (42.3971, -80.3272) -> (43.5971, -80.3272) centre (42.9971, -80.3272) ccw
  arc A1004 (38.8971, -82.5812) -> (40.0971, -82.5812) centre (39.4971, -82.5812) ccw
  arc A1005 (40.0971, -82.5812) -> (38.8971, -82.5812) centre (39.4971, -82.5812) ccw
  arc A1006 (24.547, -80.3272) -> (23.347, -80.3272) centre (23.947, -80.3272) ccw
  arc A1007 (23.347, -80.3272) -> (24.547, -80.3272) centre (23.947, -80.3272) ccw
  arc A1008 (21.047, -82.5812) -> (19.847, -82.5812) centre (20.447, -82.5812) ccw
  arc A1009 (19.847, -82.5812) -> (21.047, -82.5812) centre (20.447, -82.5812) ccw
  arc A1010 (5.497, -80.3272) -> (4.297, -80.3272) centre (4.897, -80.3272) ccw
  arc A1011 (4.297, -80.3272) -> (5.497, -80.3272) centre (4.897, -80.3272) ccw
  arc A1012 (0.797, -82.5812) -> (1.997, -82.5812) centre (1.397, -82.5812) ccw
  arc A1013 (1.997, -82.5812) -> (0.797, -82.5812) centre (1.397, -82.5812) ccw
  arc A1014 (61.4471, -23.1516) -> (62.6471, -23.1516) centre (62.0471, -23.1516) ccw
  arc A1015 (62.6471, -23.1516) -> (61.4471, -23.1516) centre (62.0471, -23.1516) ccw
  arc A1016 (57.9471, -25.4057) -> (59.1471, -25.4057) centre (58.5471, -25.4057) ccw
  arc A1017 (59.1471, -25.4057) -> (57.9471, -25.4057) centre (58.5471, -25.4057) ccw
  arc A1018 (42.3971, -42.2017) -> (43.5971, -42.2017) centre (42.9971, -42.2017) ccw
  arc A1019 (43.5971, -42.2017) -> (42.3971, -42.2017) centre (42.9971, -42.2017) ccw
  arc A1020 (40.0971, -44.4557) -> (38.8971, -44.4557) centre (39.4971, -44.4557) ccw
  arc A1021 (38.8971, -44.4557) -> (40.0971, -44.4557) centre (39.4971, -44.4557) ccw
  arc A1022 (42.3971, -23.1516) -> (43.5971, -23.1516) centre (42.9971, -23.1516) ccw
  arc A1023 (43.5971, -23.1516) -> (42.3971, -23.1516) centre (42.9971, -23.1516) ccw
  arc A1024 (40.0971, -25.4057) -> (38.8971, -25.4057) centre (39.4971, -25.4057) ccw
  arc A1025 (38.8971, -25.4057) -> (40.0971, -25.4057) centre (39.4971, -25.4057) ccw
  arc A1026 (24.547, -23.1516) -> (23.347, -23.1516) centre (23.947, -23.1516) ccw
  arc A1027 (23.347, -23.1516) -> (24.547, -23.1516) centre (23.947, -23.1516) ccw
  arc A1028 (21.047, -25.4057) -> (19.847, -25.4057) centre (20.447, -25.4057) ccw
  arc A1029 (19.847, -25.4057) -> (21.047, -25.4057) centre (20.447, -25.4057) ccw
  arc A1030 (24.547, -61.2644) -> (23.347, -61.2644) centre (23.947, -61.2644) ccw
  arc A1031 (23.347, -61.2644) -> (24.547, -61.2644) centre (23.947, -61.2644) ccw
  arc A1032 (21.047, -63.5184) -> (19.847, -63.5184) centre (20.447, -63.5184) ccw
  arc A1033 (19.847, -63.5184) -> (21.047, -63.5184) centre (20.447, -63.5184) ccw
  arc A1034 (24.547, -42.2017) -> (23.347, -42.2017) centre (23.947, -42.2017) ccw
  arc A1035 (23.347, -42.2017) -> (24.547, -42.2017) centre (23.947, -42.2017) ccw
  arc A1036 (19.847, -44.4557) -> (21.047, -44.4557) centre (20.447, -44.4557) ccw
  arc A1037 (21.047, -44.4557) -> (19.847, -44.4557) centre (20.447, -44.4557) ccw
  arc A1038 (4.297, -23.1516) -> (5.497, -23.1516) centre (4.897, -23.1516) ccw
  arc A1039 (5.497, -23.1516) -> (4.297, -23.1516) centre (4.897, -23.1516) ccw
  arc A1040 (1.997, -25.4057) -> (0.797, -25.4057) centre (1.397, -25.4057) ccw
  arc A1041 (0.797, -25.4057) -> (1.997, -25.4057) centre (1.397, -25.4057) ccw
  arc A1042 (4.297, -42.2017) -> (5.497, -42.2017) centre (4.897, -42.2017) ccw
  arc A1043 (5.497, -42.2017) -> (4.297, -42.2017) centre (4.897, -42.2017) ccw
  arc A1044 (1.997, -44.4557) -> (0.797, -44.4557) centre (1.397, -44.4557) ccw
  arc A1045 (0.797, -44.4557) -> (1.997, -44.4557) centre (1.397, -44.4557) ccw
  arc A1046 (4.297, -61.2644) -> (5.497, -61.2644) centre (4.897, -61.2644) ccw
  arc A1047 (5.497, -61.2644) -> (4.297, -61.2644) centre (4.897, -61.2644) ccw
  arc A1048 (0.797, -63.5184) -> (1.997, -63.5184) centre (1.397, -63.5184) ccw
  arc A1049 (1.997, -63.5184) -> (0.797, -63.5184) centre (1.397, -63.5184) ccw
  arc A1050 (213.8474, -61.2644) -> (215.0474, -61.2644) centre (214.4474, -61.2644) ccw
  arc A1051 (215.0474, -61.2644) -> (213.8474, -61.2644) centre (214.4474, -61.2644) ccw
  arc A1052 (211.5474, -63.5184) -> (210.3474, -63.5184) centre (210.9474, -63.5184) ccw
  arc A1053 (210.3474, -63.5184) -> (211.5474, -63.5184) centre (210.9474, -63.5184) ccw
  arc A1054 (215.0474, -42.2017) -> (213.8474, -42.2017) centre (214.4474, -42.2017) ccw
  arc A1055 (213.8474, -42.2017) -> (215.0474, -42.2017) centre (214.4474, -42.2017) ccw
  arc A1056 (211.5474, -44.4557) -> (210.3474, -44.4557) centre (210.9474, -44.4557) ccw
  arc A1057 (210.3474, -44.4557) -> (211.5474, -44.4557) centre (210.9474, -44.4557) ccw
  arc A1058 (213.8474, -23.1516) -> (215.0474, -23.1516) centre (214.4474, -23.1516) ccw
  arc A1059 (215.0474, -23.1516) -> (213.8474, -23.1516) centre (214.4474, -23.1516) ccw
  arc A1060 (210.3474, -25.4057) -> (211.5474, -25.4057) centre (210.9474, -25.4057) ccw
  arc A1061 (211.5474, -25.4057) -> (210.3474, -25.4057) centre (210.9474, -25.4057) ccw
  arc A1062 (215.0474, -80.3272) -> (213.8474, -80.3272) centre (214.4474, -80.3272) ccw
  arc A1063 (213.8474, -80.3272) -> (215.0474, -80.3272) centre (214.4474, -80.3272) ccw
  arc A1064 (211.5474, -82.5812) -> (210.3474, -82.5812) centre (210.9474, -82.5812) ccw
  arc A1065 (210.3474, -82.5812) -> (211.5474, -82.5812) centre (210.9474, -82.5812) ccw
  arc A1066 (195.9974, -42.2017) -> (194.7974, -42.2017) centre (195.3974, -42.2017) ccw
  arc A1067 (194.7974, -42.2017) -> (195.9974, -42.2017) centre (195.3974, -42.2017) ccw
  arc A1068 (192.4974, -44.4557) -> (191.2974, -44.4557) centre (191.8974, -44.4557) ccw
  arc A1069 (191.2974, -44.4557) -> (192.4974, -44.4557) centre (191.8974, -44.4557) ccw
  arc A1070 (175.1224, -4.318) -> (176.9224, -4.318) centre (176.0224, -4.318) ccw
  arc A1071 (176.9224, -4.318) -> (175.1224, -4.318) centre (176.0224, -4.318) ccw
  line L7082 (174.3823, -3.418) -> (174.3823, -5.218)
  line L7083 (172.5823, -5.218) -> (172.5823, -3.418)
  line L7084 (172.5823, -3.418) -> (174.3823, -3.418)
  line L7085 (174.3823, -5.218) -> (172.5823, -5.218)
  line L7086 (199.9454, -1.747) -> (200.3154, -1.747)
  line L7087 (200.3154, -1.505) -> (200.2654, -1.455)
  line L7088 (200.2654, -1.455) -> (199.4654, -1.455)
  line L7089 (200.2654, -2.355) -> (200.3154, -2.305)
  line L7090 (199.4654, -1.455) -> (199.4154, -1.505)
  line L7091 (200.3154, -2.077) -> (199.9454, -2.077)
  line L7092 (199.4654, -2.355) -> (200.2654, -2.355)
  line L7093 (200.3154, -2.305) -> (200.3154, -2.077)
  line L7094 (199.4154, -1.505) -> (199.4154, -2.305)
  line L7095 (200.3154, -1.747) -> (200.3154, -1.505)
  line L7096 (199.9454, -2.077) -> (199.9454, -1.747)
  line L7097 (199.4154, -2.305) -> (199.4654, -2.355)
  line L7098 (201.0554, -1.455) -> (201.0054, -1.505)
  line L7099 (201.0054, -1.505) -> (201.0054, -1.733)
  line L7100 (201.0054, -2.063) -> (201.0054, -2.305)
  line L7101 (201.3754, -1.733) -> (201.3754, -2.063)
  line L7102 (201.0054, -1.733) -> (201.3754, -1.733)
  line L7103 (201.0554, -2.355) -> (201.8554, -2.355)
  line L7104 (201.8554, -2.355) -> (201.9054, -2.305)
  line L7105 (201.8554, -1.455) -> (201.0554, -1.455)
  line L7106 (201.9054, -2.305) -> (201.9054, -1.505)
  line L7107 (201.9054, -1.505) -> (201.8554, -1.455)
  line L7108 (201.0054, -2.305) -> (201.0554, -2.355)
  line L7109 (201.3754, -2.063) -> (201.0054, -2.063)
  line L7110 (208.5746, -5.023) -> (208.3746, -5.023)
  line L7111 (208.3746, -5.023) -> (208.3746, -5.688)
  line L7112 (208.5746, -5.688) -> (208.5746, -5.023)
  line L7113 (208.3746, -5.688) -> (208.5746, -5.688)
  line L7114 (211.3744, -5.023) -> (211.1744, -5.023)
  line L7115 (211.3744, -5.688) -> (211.3744, -5.023)
  line L7116 (211.1744, -5.023) -> (211.1744, -5.688)
  line L7117 (211.1744, -5.688) -> (211.3744, -5.688)
  line L7118 (210.9744, -5.688) -> (210.9744, -5.023)
  line L7119 (210.7744, -5.023) -> (210.7744, -5.688)
  line L7120 (210.9744, -5.023) -> (210.7744, -5.023)
  line L7121 (210.7744, -5.688) -> (210.9744, -5.688)
  line L7122 (213.5745, -5.023) -> (213.5745, -5.688)
  line L7123 (213.7745, -5.023) -> (213.5745, -5.023)
  line L7124 (213.7745, -5.688) -> (213.7745, -5.023)
  line L7125 (213.5745, -5.688) -> (213.7745, -5.688)
  line L7126 (208.7744, -5.023) -> (208.7744, -5.688)
  line L7127 (208.7744, -5.688) -> (208.9744, -5.688)
  line L7128 (208.9744, -5.023) -> (208.7744, -5.023)
  line L7129 (208.9744, -5.688) -> (208.9744, -5.023)
  line L7130 (211.5745, -5.023) -> (211.5745, -5.688)
  line L7131 (211.7745, -5.688) -> (211.7745, -5.023)
  line L7132 (211.7745, -5.023) -> (211.5745, -5.023)
  line L7133 (211.5745, -5.688) -> (211.7745, -5.688)
  line L7134 (209.1744, -5.023) -> (209.1744, -5.688)
  line L7135 (209.3744, -5.688) -> (209.3744, -5.023)
  line L7136 (209.1744, -5.688) -> (209.3744, -5.688)
  line L7137 (209.3744, -5.023) -> (209.1744, -5.023)
  line L7138 (212.1745, -5.023) -> (211.9745, -5.023)
  line L7139 (211.9745, -5.688) -> (212.1745, -5.688)
  line L7140 (211.9745, -5.023) -> (211.9745, -5.688)
  line L7141 (212.1745, -5.688) -> (212.1745, -5.023)
  line L7142 (209.7745, -5.023) -> (209.5745, -5.023)
  line L7143 (209.7745, -5.688) -> (209.7745, -5.023)
  line L7144 (209.5745, -5.688) -> (209.7745, -5.688)
  line L7145 (209.5745, -5.023) -> (209.5745, -5.688)
  line L7146 (212.5746, -5.688) -> (212.5746, -5.023)
  line L7147 (212.5746, -5.023) -> (212.3746, -5.023)
  line L7148 (212.3746, -5.023) -> (212.3746, -5.688)
  line L7149 (212.3746, -5.688) -> (212.5746, -5.688)
  line L7150 (210.3746, -5.688) -> (210.5746, -5.688)
  line L7151 (210.5746, -5.023) -> (210.3746, -5.023)
  line L7152 (210.3746, -5.023) -> (210.3746, -5.688)
  line L7153 (210.5746, -5.688) -> (210.5746, -5.023)
  line L7154 (213.3744, -5.688) -> (213.3744, -5.023)
  line L7155 (213.3744, -5.023) -> (213.1744, -5.023)
  line L7156 (213.1744, -5.023) -> (213.1744, -5.688)
  line L7157 (213.1744, -5.688) -> (213.3744, -5.688)
  line L7158 (210.1745, -5.023) -> (209.9745, -5.023)
  line L7159 (209.9745, -5.023) -> (209.9745, -5.688)
  line L7160 (210.1745, -5.688) -> (210.1745, -5.023)
  line L7161 (209.9745, -5.688) -> (210.1745, -5.688)
  line L7162 (212.9744, -5.688) -> (212.9744, -5.023)
  line L7163 (212.7744, -5.023) -> (212.7744, -5.688)
  line L7164 (212.7744, -5.688) -> (212.9744, -5.688)
  line L7165 (212.9744, -5.023) -> (212.7744, -5.023)
  line L7166 (207.9994, -6.0629) -> (207.3344, -6.0629)
  line L7167 (207.3344, -6.2629) -> (207.9994, -6.2629)
  line L7168 (207.3344, -6.0629) -> (207.3344, -6.2629)
  line L7169 (207.9994, -6.2629) -> (207.9994, -6.0629)
  line L7170 (214.1495, -6.2629) -> (214.8145, -6.2629)
  line L7171 (214.8145, -6.2629) -> (214.8145, -6.0629)
  line L7172 (214.8145, -6.0629) -> (214.1495, -6.0629)
  line L7173 (214.1495, -6.0629) -> (214.1495, -6.2629)
  line L7174 (207.3344, -6.463) -> (207.3344, -6.663)
  line L7175 (207.9994, -6.463) -> (207.3344, -6.463)
  line L7176 (207.9994, -6.663) -> (207.9994, -6.463)
  line L7177 (207.3344, -6.663) -> (207.9994, -6.663)
  line L7178 (214.8145, -6.463) -> (214.1495, -6.463)
  line L7179 (214.8145, -6.663) -> (214.8145, -6.463)
  line L7180 (214.1495, -6.463) -> (214.1495, -6.663)
  line L7181 (214.1495, -6.663) -> (214.8145, -6.663)
  line L7182 (207.9994, -6.863) -> (207.3344, -6.863)
  line L7183 (207.3344, -7.063) -> (207.9994, -7.063)
  line L7184 (207.3344, -6.863) -> (207.3344, -7.063)
  line L7185 (207.9994, -7.063) -> (207.9994, -6.863)
  line L7186 (214.1495, -6.863) -> (214.1495, -7.063)
  line L7187 (214.8145, -7.063) -> (214.8145, -6.863)
  line L7188 (214.8145, -6.863) -> (214.1495, -6.863)
  line L7189 (214.1495, -7.063) -> (214.8145, -7.063)
  line L7190 (214.8145, -7.4628) -> (214.8145, -7.2628)
  line L7191 (214.8145, -7.2628) -> (214.1495, -7.2628)
  line L7192 (214.1495, -7.2628) -> (214.1495, -7.4628)
  line L7193 (214.1495, -7.4628) -> (214.8145, -7.4628)
  line L7194 (207.3344, -7.4628) -> (207.9994, -7.4628)
  line L7195 (207.9994, -7.2628) -> (207.3344, -7.2628)
  line L7196 (207.3344, -7.2628) -> (207.3344, -7.4628)
  line L7197 (207.9994, -7.4628) -> (207.9994, -7.2628)
  line L7198 (207.3344, -7.6629) -> (207.3344, -7.8629)
  line L7199 (207.3344, -7.8629) -> (207.9994, -7.8629)
  line L7200 (207.9994, -7.6629) -> (207.3344, -7.6629)
  line L7201 (207.9994, -7.8629) -> (207.9994, -7.6629)
  line L7202 (214.8145, -7.6629) -> (214.1495, -7.6629)
  line L7203 (214.1495, -7.6629) -> (214.1495, -7.8629)
  line L7204 (214.8145, -7.8629) -> (214.8145, -7.6629)
  line L7205 (214.1495, -7.8629) -> (214.8145, -7.8629)
  line L7206 (207.3344, -8.2629) -> (207.9994, -8.2629)
  line L7207 (207.9994, -8.0629) -> (207.3344, -8.0629)
  line L7208 (207.3344, -8.0629) -> (207.3344, -8.2629)
  line L7209 (207.9994, -8.2629) -> (207.9994, -8.0629)
  line L7210 (214.1495, -8.2629) -> (214.8145, -8.2629)
  line L7211 (214.8145, -8.2629) -> (214.8145, -8.0629)
  line L7212 (214.8145, -8.0629) -> (214.1495, -8.0629)
  line L7213 (214.1495, -8.0629) -> (214.1495, -8.2629)
  line L7214 (207.3344, -8.463) -> (207.3344, -8.663)
  line L7215 (207.9994, -8.463) -> (207.3344, -8.463)
  line L7216 (207.9994, -8.663) -> (207.9994, -8.463)
  line L7217 (207.3344, -8.663) -> (207.9994, -8.663)
  line L7218 (214.8145, -8.463) -> (214.1495, -8.463)
  line L7219 (214.1495, -8.463) -> (214.1495, -8.663)
  line L7220 (214.8145, -8.663) -> (214.8145, -8.463)
  line L7221 (214.1495, -8.663) -> (214.8145, -8.663)
  line L7222 (207.9994, -9.063) -> (207.9994, -8.863)
  line L7223 (207.9994, -8.863) -> (207.3344, -8.863)
  line L7224 (207.3344, -9.063) -> (207.9994, -9.063)
  line L7225 (207.3344, -8.863) -> (207.3344, -9.063)
  line L7226 (214.8145, -8.863) -> (214.1495, -8.863)
  line L7227 (214.1495, -8.863) -> (214.1495, -9.063)
  line L7228 (214.1495, -9.063) -> (214.8145, -9.063)
  line L7229 (214.8145, -9.063) -> (214.8145, -8.863)
  line L7230 (207.3344, -9.2628) -> (207.3344, -9.4628)
  line L7231 (207.9994, -9.4628) -> (207.9994, -9.2628)
  line L7232 (207.9994, -9.2628) -> (207.3344, -9.2628)
  line L7233 (207.3344, -9.4628) -> (207.9994, -9.4628)
  line L7234 (214.1495, -9.2628) -> (214.1495, -9.4628)
  line L7235 (214.8145, -9.4628) -> (214.8145, -9.2628)
  line L7236 (214.8145, -9.2628) -> (214.1495, -9.2628)
  line L7237 (214.1495, -9.4628) -> (214.8145, -9.4628)
  line L7238 (207.9994, -9.8629) -> (207.9994, -9.6629)
  line L7239 (207.3344, -9.8629) -> (207.9994, -9.8629)
  line L7240 (207.9994, -9.6629) -> (207.3344, -9.6629)
  line L7241 (207.3344, -9.6629) -> (207.3344, -9.8629)
  line L7242 (214.8145, -9.6629) -> (214.1495, -9.6629)
  line L7243 (214.1495, -9.8629) -> (214.8145, -9.8629)
  line L7244 (214.8145, -9.8629) -> (214.8145, -9.6629)
  line L7245 (214.1495, -9.6629) -> (214.1495, -9.8629)
  line L7246 (214.8145, -10.2629) -> (214.8145, -10.0629)
  line L7247 (214.1495, -10.2629) -> (214.8145, -10.2629)
  line L7248 (214.1495, -10.0629) -> (214.1495, -10.2629)
  line L7249 (214.8145, -10.0629) -> (214.1495, -10.0629)
  line L7250 (207.3344, -10.2629) -> (207.9994, -10.2629)
  line L7251 (207.9994, -10.2629) -> (207.9994, -10.0629)
  line L7252 (207.9994, -10.0629) -> (207.3344, -10.0629)
  line L7253 (207.3344, -10.0629) -> (207.3344, -10.2629)
  line L7254 (207.9994, -10.463) -> (207.3344, -10.463)
  line L7255 (207.9994, -10.663) -> (207.9994, -10.463)
  line L7256 (207.3344, -10.463) -> (207.3344, -10.663)
  line L7257 (207.3344, -10.663) -> (207.9994, -10.663)
  line L7258 (214.8145, -10.663) -> (214.8145, -10.463)
  line L7259 (214.8145, -10.463) -> (214.1495, -10.463)
  line L7260 (214.1495, -10.463) -> (214.1495, -10.663)
  line L7261 (214.1495, -10.663) -> (214.8145, -10.663)
  line L7262 (207.9994, -11.063) -> (207.9994, -10.863)
  line L7263 (207.9994, -10.863) -> (207.3344, -10.863)
  line L7264 (207.3344, -10.863) -> (207.3344, -11.063)
  line L7265 (207.3344, -11.063) -> (207.9994, -11.063)
  line L7266 (214.1495, -11.063) -> (214.8145, -11.063)
  line L7267 (214.8145, -10.863) -> (214.1495, -10.863)
  line L7268 (214.1495, -10.863) -> (214.1495, -11.063)
  line L7269 (214.8145, -11.063) -> (214.8145, -10.863)
  line L7270 (207.3344, -11.4628) -> (207.9994, -11.4628)
  line L7271 (207.9994, -11.4628) -> (207.9994, -11.2628)
  line L7272 (207.3344, -11.2628) -> (207.3344, -11.4628)
  line L7273 (207.9994, -11.2628) -> (207.3344, -11.2628)
  line L7274 (214.1495, -11.4628) -> (214.8145, -11.4628)
  line L7275 (214.1495, -11.2628) -> (214.1495, -11.4628)
  line L7276 (214.8145, -11.2628) -> (214.1495, -11.2628)
  line L7277 (214.8145, -11.4628) -> (214.8145, -11.2628)
  line L7278 (213.5745, -12.5031) -> (213.7745, -12.5031)
  line L7279 (213.7745, -11.8381) -> (213.5745, -11.8381)
  line L7280 (213.5745, -11.8381) -> (213.5745, -12.5031)
  line L7281 (213.7745, -12.5031) -> (213.7745, -11.8381)
  line L7282 (210.9744, -12.5031) -> (210.9744, -11.8381)
  line L7283 (210.7744, -12.5031) -> (210.9744, -12.5031)